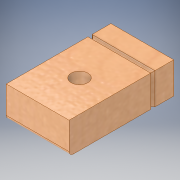
# Autodesk Inventor part: peg_half
Saved by Autodesk Inventor 2019 (Build 230136000, 136)
## iProperties
Created: 2019-12-28
Part Number: peg_half
Material: Клен
Document SubType Name: Modeling
Designer: stepa
Density: 0.705 g/cm^3
Appearance: Клен — массив — натуральный — с умеренным глянцем
Author: stepa
Autodesk Inventor part; units mm, degrees
ref_plane "YZ Plane" through (0, 0, 0) normal (1, 0, 0) x (0, 1, 0)
ref_plane "XZ Plane" through (0, 0, 0) normal (0, 1, 0) x (-1, 0, 0)
ref_plane "XY Plane" through (0, 0, 0) normal (0, 0, 1) x (1, 0, 0)
sketch "Эскиз1" plane through (0, 0, 0) normal (0, 1, 0) x (-1, 0, 0)
  line L0 (0, 0) -> (30, 0)
  line L1 (30, 0) -> (30, -50)
  line L2 (30, -50) -> (0, -50)
  line L3 (0, -50) -> (0, 0)
  dimension "d0" = 30
  dimension "d1" = 50
  constraints: 8 end point, 2 parallel, 1 horizontal, 1 perpendicular
  measures "d0" distance of L1.end L2.end
  measures "d1" distance of L0.end L1.end
extrude "Выдавливание1" add sketch "Эскиз1" along normal blind 15
fillet "Сопряжение1" radius 2 1 edges at (-15, 0, 0)
sketch "Эскиз2" plane through (0, 15, 0) normal (0, 1, 0) x (1, 0, 0)
  line L0 (-30, 0) -> (0, 0) projected
  point P0 (-15, 20)
  point P1 (-15, 0)
  dimension "d5" = 20
  constraints: 1 midpoint, 1 vertical alignment
  measures "d5" distance from line of L0 point (-15, 20)
hole "Отверстие1" at (-15, 15, -20) direction (0, -1, 0) diameter 8 end through all
sketch "Эскиз3" plane through (0, 15, 0) normal (0, 1, 0) x (1, 0, 0)
  line L0 (-30, 0) -> (0, 0) projected
  circle A0 centre (-15, 20) radius 4 projected
  line L1 (-30, 0) -> (0, 0) projected
  line L2 (0, 0) -> (0, 50) projected
  line L3 (0, 50) -> (-30, 50) projected
  line L4 (-30, 50) -> (-30, 0) projected
  line L5 (-30, 50) -> (-30, 0) projected
  line L6 (0, 0) -> (0, 50) projected
  point P0 (-30, 40)
  point P1 (0, 40)
  dimension "d13" = 40
  constraints: 2 point on line, 1 horizontal alignment
  measures "d13" distance from line of L0 point (-30, 40)
hole "Отверстие2" at (-30, 15, -40) at (0, 15, -40) direction (0, -1, 0) diameter 2 end through all
sketch "Эскиз4" plane through (0, 2, 0) normal (1, 0, 0) x (0, 0, -1)
  line L0 (41, 13) -> (41, -2) projected
  line L1 (39, 13) -> (41, 13) projected
  line L2 (39, -2) -> (39, 13) projected
  line L3 (41, -2) -> (39, -2) projected
  line L4 (39, 13) -> (41, 13) projected
  point P0 (0, -2)
  point P1 (40, 13)
  constraints: 1 midpoint
hole "Отверстие3" at (0, 15, -40) direction (-1, 0, 0) diameter 2 end through all
